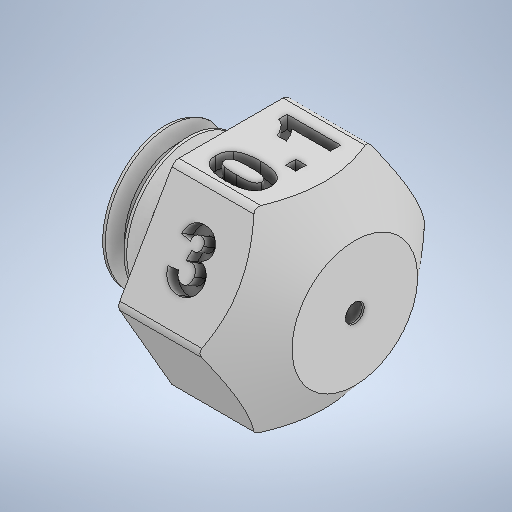
# Autodesk Inventor part: Part1
Saved by Autodesk Inventor 2025.2 (Build 292293000, 293)
## iProperties
Created: 2026-03-09
Part Number: Part1
Material: Generic
Document SubType Name: Modeling
Designer: Simon
Density: 1 g/cm^3
Appearance: Default
Author: Simon
Autodesk Inventor part; units mm, degrees
ref_plane "YZ Plane" through (0, 0, 0) normal (1, 0, 0) x (0, 1, 0)
ref_plane "XZ Plane" through (0, 0, 0) normal (0, 1, 0) x (-1, 0, 0)
ref_plane "XY Plane" through (0, 0, 0) normal (0, 0, 1) x (1, 0, 0)
sketch "Sketch1" plane through (0, 0, 0) normal (0, 0, 1) x (1, 0, 0)
  line L0 (0, 0) -> (0, 1.25)
  line L1 (0, 1.25) -> (50, 1.25)
  line L2 (0, 0) -> (0, 0.336)
  line L3 (0, 0.336) -> (50, 0.336)
  line L4 (0, 0) -> (0, 0.3513)
  line L5 (0, 0.3513) -> (50, 0.3513)
  line L6 (0, 0) -> (0, 2.5)
  line L7 (0, 2.5) -> (2.5, 2.5)
  line L8 (2.5, 2.5) -> (2.5, 1.25)
  line L9 (2.5, 1.25) -> (2.5, 4.25)
  line L10 (2.5, 1.25) -> (6.7109, 1.25) construction
  line L11 (2.5, 4.25) -> (5.5, 4.25)
  line L12 (5.5, 4.25) -> (5.5, 1.25)
  line L13 (5.5, 1.25) -> (7.0831, 0.336)
  line L14 (5.5, 1.25) -> (9.25, 1.25) construction
  line L15 (7.0831, 0.336) -> (7.1405, 0.3513)
  line L16 (7.0831, 0.336) -> (7.1425, 0.336) construction
  line L17 (7.1405, 0.3513) -> (7.1405, 2.3513)
  line L18 (7.1405, 2.3513) -> (5.5, 4.25)
  line L19 (0, 0) -> (50, 0)
  dimension "d0" = 1.25
  dimension "d1" = 50
  dimension "d2" = 0.336
  dimension "d3" = 0.3513
  dimension "d4" = 2.5
  dimension "d5" = 2.5
  dimension "d6" = 3
  dimension "d8" = 3
  dimension "d9" = 30
  dimension "d10" = 15
  dimension "d12" = 2
  dimension "d13" = 50
  constraints: 40 end point, 7 perpendicular, 7 point on line, 5 horizontal, 2 vertical, 1 equal length
  measures "d0" distance of L0.start L0.end
  measures "d1" distance of L0.end L1.end
  measures "d2" distance of L0.start L2.end
  measures "d3" distance of L0.start L4.end
  measures "d4" distance of L0.start L6.end
  measures "d5" distance of L6.end L7.end
  measures "d6" distance of L8.end L9.end
  measures "d8" distance of L9.end L11.end
  measures "d9" angle of L13 L14
  measures "d10" angle of L16 L15
  measures "d12" distance of L15.end L17.end
  measures "d13" distance of L0.start L19.end
revolve "Revolution1" add sketch "Sketch1" angle 360 about axis through (0, 0, 0) along (1, 0, 0) contours L13 L5 L15 | L6 L7 L8 L1 | L13 L1 L17 L5 | L8 L9 L11 L12 L1 | L12 L18 L17 L1
sketch "Sketch2" plane through (2.5, 0, 0) normal (-1, 0, 0) x (0, 0, 1)
  circle A0 centre (0, 0) radius 4.25 projected
  line L0 (-4.25, 0) -> (4.25, 0)
  circle A1 centre (0, 0) radius 0.336 projected
  line L1 (4.25, 0) -> (2.125, -3.6806)
  line L2 (2.125, -3.6806) -> (-2.125, -3.6806)
  line L3 (-2.125, -3.6806) -> (-4.25, 0)
  line L4 (-4.25, 0) -> (-2.125, 3.6806)
  line L5 (-2.125, 3.6806) -> (2.125, 3.6806)
  line L6 (2.125, 3.6806) -> (4.25, 0)
  circle A2 centre (0, 0) radius 1.25
  constraints: 14 end point, 2 coincident, 2 point on circle, 1 centre point, 1 horizontal, 13 other
extrude "Extrusion1" cut sketch "Sketch2" against normal through all contours L6 A0 | A0 L1 | L5 A0 | A0 L2 | L4 A0 | A0 L3
fillet "Fillet1" radius 0.3 6 edges at (4, 3.6806, 2.125) (4, 3.6806, -2.125) (4, 0, -4.25) (4, -3.6806, -2.125) (4, -3.6806, 2.125) (4, 0, 4.25)
sketch "Sketch3" plane through (0, 0, 0) normal (0, 0, 1) x (1, 0, 0)
  line L0 (-0.35, 1.8938) -> (0.45, 1.8938)
  line L1 (-0.35, 1.8938) -> (0.05, 2.5866)
  line L2 (-0.35, 1.8938) -> (0.45, 1.8938) construction
  line L3 (0.05, 2.5866) -> (0.45, 1.8938)
  line L4 (-0.0972, 3.8266) -> (0.7028, 3.8266) construction
  line L5 (0.05, 2.5866) -> (0.05, 1.8938)
  line L6 (0.05, 1.8938) -> (0.05, 2.0671)
  line L7 (0.05, 2.0671) -> (0.45, 2.0671)
  line L8 (0.45, 2.0671) -> (-0.35, 2.0671)
  line L9 (0.05, 2.5866) -> (0.05, 2.5)
  line L10 (0.05, 2.5) -> (0.45, 2.5)
  line L11 (0.45, 2.5) -> (-0.35, 2.5)
  line L12 (-0.35, 1.8938) -> (-1.15, 1.8938)
  line L13 (0.05, 2.5866) -> (-0.75, 2.5866)
  line L14 (-0.75, 2.5866) -> (-1.15, 1.8938)
  line L15 (-0.35, 1.8938) -> (-0.75, 2.5866)
  line L16 (-0.35, 2.0671) -> (-1.15, 2.0671)
  line L17 (-0.35, 2.5) -> (-0.8, 2.5)
  line L18 (-0.75, 2.5866) -> (-0.75, 1.8938)
  line L19 (-0.35, 1.8938) -> (-0.35, 1.9938)
  circle A0 centre (-0.35, 2.0938) radius 0.1
  line L20 (-0.4077, 1.9938) -> (-0.2923, 1.9938)
  line L21 (0, 2.5) -> (2.5, 2.5) projected
  line L22 (0, 2.5) -> (-0.7, 2.5)
  line L23 (-0.7, 2.5) -> (-0.4366, 2.0438)
  line L24 (-0.4366, 2.0438) -> (-0.2634, 2.0438)
  line L25 (-0.2634, 2.0438) -> (0, 2.5)
  circle A1 centre (-0.35, 2.0938) radius 0.1
  point P0 (0, 0)
  point P1 (0, 2.5)
  dimension "d18" = 0.8
  dimension "d19" = 60
  dimension "d20" = 60
  dimension "d21" = 0.1732
  dimension "d22" = 0.0866
  dimension "d23" = 0.8
  dimension "d24" = 0.1
  dimension "d25" = 0.8
  constraints: 50 end point, 13 point on line, 7 horizontal, 4 tangent, 3 midpoint, 2 centre point, 2 equal length, 2 perpendicular, 2 point on circle, 1 coincident, 1 collinear, 1 concentric, 1 parallel, 1 vertical
  measures "d18" distance of L2.start L0.end
  measures "d19" angle of L2 L1
  measures "d20" angle of L3 L4
  measures "d21" distance of L6.start L7.start
  measures "d22" distance of L3.start L10.start
  measures "d23" distance of L2.start L12.end
  measures "d24" distance of L2.start L19.end
  measures "d25" distance between parallel lines of L5 L18
coil "Coil1" sketch "Sketch3" operation cut axis through (-10, 0, 0) along (1, 0, 0) pitch 0.8 turns 4 hand right contours A0 L24 | L24 L15 L16 L8 L1 | A0 L15 L17 L11 L1 | L8 L16 A0
extrude "Extrusion2" add sketch "Sketch2" against normal blind 3 contours L1 L2 L3 L0 A2 | L0 A2 L4 L5 L6
fillet "Fillet2" radius 0.3 6 edges at (4, 3.6806, -2.125) (4, 3.6806, 2.125) (4, 0, 4.25) (4, -3.6806, 2.125) (4, -3.6806, -2.125) (4, 0, -4.25)
sketch "Sketch4" plane through (2.5, 3.6806, 1.9518) normal (0, 1, 0) x (1, 0, 0)
  line L0 (0.6024, 0.0215) -> (0.6024, 3.9041) construction
  line L1 (0.6024, 3.9041) -> (2.6436, 3.9041) construction
  line L2 (2.6436, 3.9041) -> (2.6436, 0.0215) construction
  line L3 (2.6436, 0.0215) -> (0.6024, 0.0215) construction
  spline S0 degree 2 poles (0.6024, 0.7882) (0.6024, 1.0794) (0.8098, 1.2425) knots 0 0 0 1 1 1
  spline S1 degree 2 poles (0.8098, 1.2425) (1.0552, 1.4376) (1.6238, 1.4376) knots 0 0 0 1 1 1
  spline S2 degree 2 poles (1.6238, 1.4376) (2.1909, 1.4376) (2.4393, 1.241) knots 0 0 0 1 1 1
  spline S3 degree 2 poles (2.4393, 1.241) (2.6436, 1.0794) (2.6436, 0.7882) knots 0 0 0 1 1 1
  spline S4 degree 2 poles (2.6436, 0.7882) (2.6436, 0.4955) (2.1954, 0.1388) (1.6192, 0.1388) knots 0 0 0 1 2 2 2
  spline S5 degree 2 poles (1.6192, 0.1388) (1.0552, 0.1388) (0.8067, 0.3355) knots 0 0 0 1 1 1
  spline S6 degree 2 poles (0.8067, 0.3355) (0.6024, 0.4971) (0.6024, 0.7882) knots 0 0 0 1 1 1
  spline S7 degree 2 poles (0.921, 0.7882) (0.921, 0.7181) (1.0095, 0.6099) (1.1238, 0.5794) knots 0 0 0 1 2 2 2
  spline S8 degree 2 poles (1.1238, 0.5794) (1.2717, 0.5398) (1.6238, 0.5398) knots 0 0 0 1 1 1
  spline S9 degree 2 poles (1.6238, 0.5398) (1.9744, 0.5398) (2.2381, 0.6114) (2.325, 0.7181) (2.325, 0.7882) knots 0 0 0 1 2 3 3 3
  spline S10 degree 2 poles (2.325, 0.7882) (2.325, 0.8584) (2.2366, 0.9666) (2.1223, 0.9971) knots 0 0 0 1 2 2 2
  spline S11 degree 2 poles (2.1223, 0.9971) (1.9744, 1.0367) (1.6238, 1.0367) knots 0 0 0 1 1 1
  spline S12 degree 2 poles (1.6238, 1.0367) (1.2717, 1.0367) (1.0095, 0.9651) (0.921, 0.8584) (0.921, 0.7882) knots 0 0 0 1 2 3 3 3
  line L4 (2.6101, 1.7745) -> (2.2259, 1.7745)
  line L5 (2.2259, 1.7745) -> (2.2259, 2.1587)
  line L6 (2.2259, 2.1587) -> (2.6101, 2.1587)
  line L7 (2.6101, 2.1587) -> (2.6101, 1.7745)
  line L8 (2.6101, 3.4513) -> (2.6101, 3.0672)
  line L9 (2.6101, 3.0672) -> (1.1665, 3.0672)
  spline S13 degree 2 poles (1.1665, 3.0672) (1.3616, 2.8568) (1.4561, 2.5718) knots 0 0 0 1 1 1
  line L10 (1.4561, 2.5718) -> (1.1085, 2.5718)
  spline S14 degree 2 poles (1.1085, 2.5718) (1.0598, 2.7227) (0.7854, 3.0748) (0.6024, 3.1404) knots 0 0 0 1 2 2 2
  line L11 (0.6024, 3.1404) -> (0.6024, 3.4513)
  line L12 (0.6024, 3.4513) -> (2.6101, 3.4513)
  point P0 (-2.5, 1.9518)
  constraints: 2 other
extrude "Extrusion3" cut sketch "Sketch4" against normal blind 0.5
sketch "Sketch5" plane through (2.5, 0.15, 4.1634) normal (0, 0.5, 0.866) x (1, 0, 0)
  line L0 (0.9542, 2.9752) -> (2.5076, 2.9752) construction
  line L1 (2.5076, 2.9752) -> (2.5076, 0.9675) construction
  line L2 (2.5076, 0.9675) -> (0.9542, 0.9675) construction
  line L3 (0.9542, 0.9675) -> (0.9542, 2.9752) construction
  line L4 (1.0594, 1.4996) -> (1.4299, 1.5453)
  spline S0 degree 2 poles (1.4299, 1.5453) (1.4481, 1.4035) (1.6036, 1.2526) (1.7134, 1.2526) knots 0 0 0 1 2 2 2
  spline S1 degree 2 poles (1.7134, 1.2526) (1.8323, 1.2526) (1.9939, 1.4325) (1.9939, 1.5849) knots 0 0 0 1 2 2 2
  spline S2 degree 2 poles (1.9939, 1.5849) (1.9939, 1.7297) (1.8399, 1.8989) (1.7286, 1.8989) knots 0 0 0 1 2 2 2
  spline S3 degree 2 poles (1.7286, 1.8989) (1.6555, 1.8989) (1.5533, 1.87) knots 0 0 0 1 1 1
  line L5 (1.5533, 1.87) -> (1.596, 2.1825)
  spline S4 degree 2 poles (1.596, 2.1825) (1.7515, 2.1779) (1.9146, 2.3212) (1.9146, 2.4401) knots 0 0 0 1 2 2 2
  spline S5 degree 2 poles (1.9146, 2.4401) (1.9146, 2.5407) (1.7942, 2.6596) (1.6951, 2.6596) knots 0 0 0 1 2 2 2
  spline S6 degree 2 poles (1.6951, 2.6596) (1.596, 2.6596) (1.4573, 2.5239) (1.4421, 2.3928) knots 0 0 0 1 2 2 2
  line L6 (1.4421, 2.3928) -> (1.0884, 2.4523)
  spline S7 degree 2 poles (1.0884, 2.4523) (1.125, 2.6337) (1.2744, 2.8517) (1.5396, 2.9752) (1.7058, 2.9752) knots 0 0 0 1 2 3 3 3
  spline S8 degree 2 poles (1.7058, 2.9752) (1.9878, 2.9752) (2.1585, 2.7953) knots 0 0 0 1 1 1
  spline S9 degree 2 poles (2.1585, 2.7953) (2.2988, 2.6489) (2.2988, 2.463) knots 0 0 0 1 1 1
  spline S10 degree 2 poles (2.2988, 2.463) (2.2988, 2.2008) (2.0106, 2.0438) knots 0 0 0 1 1 1
  spline S11 degree 2 poles (2.0106, 2.0438) (2.1829, 2.0072) (2.3872, 1.7496) (2.3872, 1.5682) knots 0 0 0 1 2 2 2
  spline S12 degree 2 poles (2.3872, 1.5682) (2.3872, 1.3044) (2.003, 0.934) (1.7164, 0.934) knots 0 0 0 1 2 2 2
  spline S13 degree 2 poles (1.7164, 0.934) (1.4451, 0.934) (1.0884, 1.2465) (1.0594, 1.4996) knots 0 0 0 1 2 2 2
  point P0 (-2.5, 1.9518)
  constraints: 2 other
extrude "Extrusion4" cut sketch "Sketch5" against normal blind 0.5
body "Solid1"
